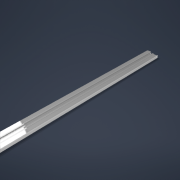
# Autodesk Inventor part: Rail_TypeA
Saved by Autodesk Inventor 2021.2 (Build 252289000, 289)
## iProperties
Created: 2021-06-16
Part Number: Rail_TypeA
Material: Aluminum
Document SubType Name: Modeling
Designer: joanh
Density: 2.7 g/cm^3
Appearance: Aluminum - Polished
Author: joanh
Autodesk Inventor part; units mm, degrees
ref_plane "YZ Plane" through (0, 0, 0) normal (1, 0, 0) x (0, 1, 0)
ref_plane "XZ Plane" through (0, 0, 0) normal (0, 1, 0) x (-1, 0, 0)
ref_plane "XY Plane" through (0, 0, 0) normal (0, 0, 1) x (1, 0, 0)
sketch "Rail_Sketch" plane through (0, 0, 0) normal (0, 0, 1) x (1, 0, 0)
  arc A0 (-1.9596, 1) -> (-1.9596, -1) centre (0, 0) ccw construction
  line L0 (-13.8, -5) -> (-11, -5) construction
  line L1 (16.5, -5) -> (16.5, 2.5)
  line L2 (16.5, 5) -> (-3.3, 5) construction
  line L3 (-13.8, 5) -> (-13.8, 3.3)
  line L4 (-13.8, 3.3) -> (-11, 3.3)
  line L5 (-11, 3.3) -> (-11, 1.6)
  line L6 (-11, 1.6) -> (-9.5, 1.6)
  line L7 (-5, 1.6) -> (-5, -1.6)
  line L8 (-5, -1.6) -> (-7, -1.6)
  line L9 (-9.5, 3) -> (-7, 3)
  line L10 (-7, 3) -> (-7, 1.6)
  line L11 (-7, -3) -> (-9.5, -3)
  line L12 (-9.5, -3) -> (-9.5, -1.6)
  line L13 (-9.5, 1.6) -> (-7, 1.6) construction
  line L14 (-7, 1.6) -> (-5, 1.6)
  line L15 (-7, 1.6) -> (-7, -1.6) construction
  line L16 (-7, -1.6) -> (-7, -3)
  line L17 (-7, -1.6) -> (-9.5, -1.6) construction
  line L18 (-9.5, -1.6) -> (-11, -1.6)
  line L19 (-9.5, -1.6) -> (-9.5, 1.6) construction
  line L20 (-9.5, 1.6) -> (-9.5, 3)
  line L21 (-11, 1.6) -> (-11, -1.6) construction
  line L22 (-11, -1.6) -> (-11, -2.2)
  line L23 (-11, -5) -> (-6, -5)
  line L24 (-3.3, 5) -> (-3.3, 4.2)
  line L25 (-3.3, 4.2) -> (-4.5, 4.2)
  line L26 (-4.5, 4.2) -> (-4.5, 2.5)
  line L27 (-13.8, 3.3) -> (-13.8, -5) construction
  line L28 (-3.3, 5) -> (-13.8, 5)
  line L29 (16.5, 2.5) -> (16.5, 5) construction
  line L30 (-3, 1) -> (-1.9596, 1)
  line L31 (3, 1) -> (3, -1)
  line L32 (3, -1) -> (1.9596, -1)
  line L33 (-3, -1) -> (-3, 1)
  line L34 (-3, 1) -> (3, -1) construction
  line L35 (3, 1) -> (-3, -1) construction
  line L36 (1.6, -2.5) -> (-1.6, -2.5)
  line L37 (-1.6, -2.5) -> (-1.6, -1.51)
  line L38 (-1.6, 2.5) -> (1.6, 2.5) construction
  line L39 (1.6, 2.5) -> (1.6, 1.51)
  line L40 (1.6, -2.5) -> (-1.6, 2.5) construction
  line L41 (-1.6, -2.5) -> (1.6, 2.5) construction
  line L42 (-1.9596, 1) -> (1.9596, 1) construction
  line L43 (1.9596, 1) -> (3, 1)
  line L44 (1.9596, -1) -> (-1.9596, -1) construction
  line L45 (-1.9596, -1) -> (-3, -1)
  line L46 (-1.6, 1.51) -> (-1.6, 2.5)
  line L47 (1.6, 1.51) -> (1.6, -1.51) construction
  line L48 (1.6, -1.51) -> (1.6, -2.5)
  line L49 (-1.6, -1.51) -> (-1.6, 1.51) construction
  arc A1 (-1.6, 1.51) -> (-1.9596, 1) centre (0, 0) ccw
  arc A2 (1.6, 1.51) -> (-1.6, 1.51) centre (0, 0) ccw construction
  arc A3 (1.9596, 1) -> (1.6, 1.51) centre (0, 0) ccw
  arc A4 (-1.6, -1.51) -> (1.6, -1.51) centre (0, 0) ccw construction
  arc A5 (-1.9596, -1) -> (-1.6, -1.51) centre (0, 0) ccw
  arc A6 (1.6, -1.51) -> (1.9596, -1) centre (0, 0) ccw
  arc A7 (1.9596, -1) -> (1.9596, 1) centre (0, 0) ccw construction
  line L50 (-4.5, 2.5) -> (-1.6, 2.5)
  line L51 (16.5, 2.5) -> (14.8, 2.5)
  line L52 (-11, -4.4) -> (-10.7, -4.4)
  line L53 (-10.7, -4.4) -> (-10.7, -2.2)
  line L54 (-10.7, -2.2) -> (-11, -2.2)
  line L55 (-11, -2.2) -> (-11, -4.4) construction
  line L56 (-11, -4.4) -> (-11, -5)
  line L57 (-6, -5) -> (-6, -4.5)
  line L58 (-6, -4.5) -> (4, -4.5)
  line L59 (4, -4.5) -> (4, -5)
  line L60 (4, -5) -> (6.8, -5)
  line L61 (-6, -5) -> (4, -5) construction
  line L62 (10, 2.5) -> (10, -5) construction
  line L63 (14.8, 2.5) -> (14.8, 1)
  line L64 (14.8, 1) -> (5.2, 1)
  line L65 (5.2, 1) -> (5.2, 2.5)
  line L66 (5.2, 2.5) -> (1.6, 2.5)
  line L67 (14.8, 2.5) -> (5.2, 2.5) construction
  line L68 (13.2, -5) -> (13.2, -3.5)
  line L69 (13.2, -3.5) -> (14.8, -3.5)
  line L70 (14.8, -3.5) -> (14.8, -1.5)
  line L71 (14.8, -1.5) -> (5.2, -1.5)
  line L72 (5.2, -1.5) -> (5.2, -3.5)
  line L73 (5.2, -3.5) -> (6.8, -3.5)
  line L74 (6.8, -3.5) -> (6.8, -5)
  line L75 (6.8, -5) -> (13.2, -5) construction
  line L76 (13.2, -5) -> (16.5, -5)
  dimension "d55" = 4.4
  dimension "d56" = 10
  dimension "d57" = 5
  dimension "d58" = 13.8
  dimension "d59" = 30.3
  dimension "d60" = 1.7
  dimension "d61" = 2.8
  dimension "d62" = 6
  dimension "d63" = 3.2
  dimension "d64" = 1.6
  dimension "d65" = 2.5
  dimension "d66" = 6
  dimension "d67" = 1.5
  dimension "d68" = 3
  dimension "d69" = 0.8
  dimension "d70" = 1.2
  dimension "d71" = 1.7
  dimension "d72" = 10.5
  dimension "d74" = 6
  dimension "d75" = 2
  dimension "d76" = 3.2
  dimension "d77" = 5
  dimension "d78" = 0.3
  dimension "d79" = 2.2
  dimension "d80" = 0.6
  dimension "d81" = 0.5
  dimension "d82" = 10
  dimension "d83" = 5
  dimension "d84" = 6.5
  dimension "d85" = 1.5
  dimension "d86" = 9.6
  dimension "d87" = 1.7
  dimension "d88" = 1.5
  dimension "d89" = 2
  dimension "d90" = 6.4
  dimension "d91" = 3.2
  dimension "d92" = 4.8
  dimension "d93" = 9.6
  constraints: 154 end point, 93 perpendicular, 60 parallel, 29 point on circle, 15 horizontal, 8 centre point, 7 point on line, 6 midpoint, 1 coincident, 1 vertical
  measures "d55" diameter of A0
  measures "d56" distance between parallel lines of L0 L2
  measures "d57" distance from line of L0 point (0, 0)
  measures "d58" distance from line of L3 point (0, 0)
  measures "d59" distance between parallel lines of L1 L3
  measures "d60" distance between parallel lines of L4 L2
  measures "d61" distance between parallel lines of L3 L5
  measures "d62" distance of L7.end L18.end
  measures "d63" distance of L7.start L7.end
  measures "d64" distance from line of point (0, 0) L6
  measures "d65" distance of L11.start L11.end
  measures "d66" distance of L9.end L11.start
  measures "d67" distance between parallel lines of L5 L12
  measures "d68" distance from line of A0.centre L9
  measures "d69" distance of L2.end L24.end
  measures "d70" distance of L24.end L25.end
  measures "d71" distance of L25.end L26.end
  measures "d72" distance between parallel lines of L3 L24
  measures "d74" distance of L31.end L33.start
  measures "d75" distance of L31.start L31.end
  measures "d76" distance of L38.start L38.end
  measures "d77" distance of L36.end L38.start
  measures "d78" distance of L52.start L52.end
  measures "d79" distance of L52.end L53.end
  measures "d80" distance between parallel lines of L23 L52
  measures "d81" distance of L23.end L57.end
  measures "d82" distance of L57.end L58.end
  measures "d83" distance between parallel lines of L56 L57
  measures "d84" distance between parallel lines of L1 L62
  measures "d85" distance of L51.end L63.end
  measures "d86" distance of L63.end L64.end
  measures "d87" distance between parallel lines of L1 L63
  measures "d88" distance of L68.start L68.end
  measures "d89" distance of L69.end L70.end
  measures "d90" distance between parallel lines of L68 L74
  measures "d91" distance between parallel lines of L62 L74
  measures "d92" distance between parallel lines of L62 L72
  measures "d93" distance between parallel lines of L70 L72
extrude "Extrusion1" add sketch "Rail_Sketch" against normal blind 426.72
fillet "Rad_0.5 mm Fillet" radius 0.5 4 edges at (6.8, -5, -213.36) (13.2, -5, -213.36) (14.8, 2.5, -213.36) (5.2, 2.5, -213.36)
fillet "Rad_1 mm Fillet" radius 1 1 edges at (-13.8, 5, -213.36)
fillet "Rad_0.8 mm Fillet" radius 0.8 1 edges at (-3.3, 5, -213.36)
fillet "Rad_0.1 mm Fillet" radius 0.1 41 edges at (16.5, -5, -213.36) (16.5, 2.5, -213.36) (6.8, -3.5, -213.36) (13.2, -3.5, -213.36) (14.8, -3.5, -213.36) (14.8, -1.5, -213.36) (5.2, -1.5, -213.36) (5.2, -3.5, -213.36) (14.8, 1, -213.36) (5.2, 1, -213.36) (1.6, 2.5, -213.36) (-1.6, 2.5, -213.36) (3, 1, -213.36) (3, -1, -213.36) (1.6, -2.5, -213.36) (-1.6, -2.5, -213.36) (-3, -1, -213.36) (-3, 1, -213.36) (-4.5, 2.5, -213.36) (-4.5, 4.2, -213.36) (-13.8, 3.3, -213.36) (-11, 3.3, -213.36) (-11, 1.6, -213.36) (-9.5, 1.6, -213.36) (-9.5, 3, -213.36) (-7, 3, -213.36) (-7, 1.6, -213.36) (-5, 1.6, -213.36) (-5, -1.6, -213.36) (-7, -1.6, -213.36) (-7, -3, -213.36) (-9.5, -3, -213.36) (-9.5, -1.6, -213.36) (-11, -1.6, -213.36) (-11, -2.2, -213.36) (-11, -4.4, -213.36) (-11, -5, -213.36) (-6, -5, -213.36) (-6, -4.5, -213.36) (4, -4.5, -213.36) (4, -5, -213.36)
equation "\"d64\" = 0.5 * d63"
equation "\"d68\" = 0.5 * d66"
equation "\"d91\" = 0.5 * d90"
equation "\"d92\" = 0.5 * d86"
equation "\"d93\" = d86"
body "Solid1"
